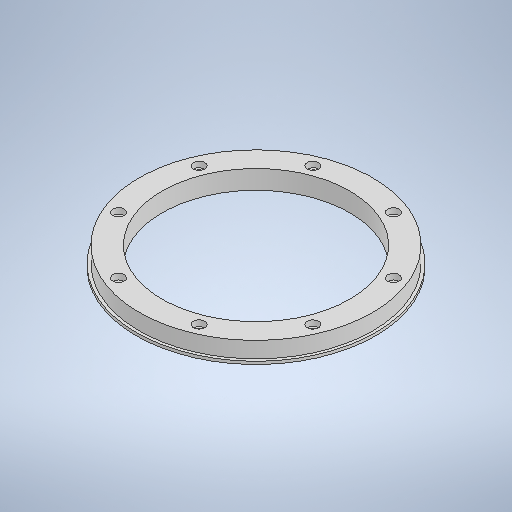
# Autodesk Inventor part: DMF 01 32 Барабан Опорное кольцо КОРМА v2.1
Saved by Autodesk Inventor 2026.2 (Build 302298000, 298)
## iProperties
Created: 2024-04-28
Part Number: DMF 01 32 Барабан Опорное кольцо КОРМА v2.1
Material: Generic
Document SubType Name: Sheet Metal
Designer: admin
Density: 1 g/cm^3
Appearance: Default
Stock Number: Опорное_Кольцо_Корма
Sheet Metal Rule: Default
Author: pokla
Autodesk Inventor part; units mm, degrees
ref_plane "YZ Plane" through (0, 0, 0) normal (1, 0, 0) x (0, 1, 0)
ref_plane "XZ Plane" through (0, 0, 0) normal (0, 1, 0) x (-1, 0, 0)
ref_plane "XY Plane" through (0, 0, 0) normal (0, 0, 1) x (1, 0, 0)
sketch "Sketch5" plane through (0, 0, 0) normal (0, 0, 1) x (1, 0, 0)
  line L0 (0, 0) -> (0, 33)
  line L1 (164, 0) -> (164, 33)
  line L2 (164, 33) -> (204, 33)
  line L3 (204, 33) -> (204, 5)
  line L4 (204, 5) -> (209, 5)
  line L5 (209, 5) -> (209, 0)
  line L6 (209, 0) -> (164, 0)
  point P0 (186.5, 0)
  dimension "d16" = 328
  dimension "d17" = 408
  dimension "d19" = 28
  dimension "d20" = 5
  dimension "d21" = 5
  constraints: 14 end point, 5 perpendicular, 2 vertical, 1 horizontal alignment, 1 midpoint, 1 point on line
  measures "d16" diameter of L1 L0
  measures "d17" diameter of L3 L0
  measures "d19" distance of L2.end L3.end
  measures "d20" distance of L4.end L5.end
  measures "d21" distance between parallel lines of L5 L3
revolve "Revolution1" add sketch "Sketch5" angle 360 about axis through (0, 0, 0) along (0, 1, 0)
sketch "Sketch6" plane through (0, 33, 0) normal (0, 1, 0) x (1, 0, 0)
  circle A0 centre (0, 0) radius 184
  line L0 (0, 0) -> (-70.4138, 169.9938)
  line L1 (0, 0) -> (0, 184)
  dimension "d23" = 368
  dimension "d34" = 22.5
  constraints: 4 end point, 2 point on circle, 1 centre point, 1 coincident, 1 vertical
  measures "d23" diameter of A0
  measures "d34" angle of L0 L1
hole "Hole1" at (-70.4138, 33, -169.9938) direction (0, -1, 0) diameter 11 end through all counterbore diameter 20 counterbore depth 10
pattern_circular "Circular Pattern2" count 8 over 360 about axis through (0, -10, 0) along (0, 1, 0) of "Hole1"
equation "\"d29\" = Thickness"
equation "\"Thickness\" = 40"
body "Solid2"
